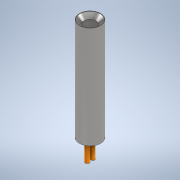
# Autodesk Inventor part: Heater630W
Saved by Autodesk Inventor 2020 (Build 240168000, 168)
## iProperties
Created: 2020-06-17
Part Number: Heater630W
Material: Steel, Alloy
Document SubType Name: Modeling
Designer: Juan
Density: 7.73 g/cm^3
Appearance: Semi-Polished
Author: Juan
Autodesk Inventor part; units mm, degrees
ref_plane "YZ Plane" through (0, 0, 0) normal (1, 0, 0) x (0, 1, 0)
ref_plane "XZ Plane" through (0, 0, 0) normal (0, 1, 0) x (-1, 0, 0)
ref_plane "XY Plane" through (0, 0, 0) normal (0, 0, 1) x (1, 0, 0)
sketch "Sketch1" plane through (0, 0, 0) normal (0, 1, 0) x (-1, 0, 0)
  circle A0 centre (0, 0) radius 7.9375
  dimension "d0" = 15.875
  constraints: 1 centre point, 1 coincident
  measures "d0" diameter of A0
extrude "Extrusion1" add sketch "Sketch1" along normal blind 76.2
sketch "Sketch2" plane through (0, 76.2, 0) normal (0, 1, 0) x (1, 0, 0)
  circle A0 centre (0, 0) radius 4.5
  dimension "d3" = 9
  constraints: 1 centre point, 1 coincident
  measures "d3" diameter of A0
extrude "Extrusion2" cut sketch "Sketch2" against normal blind 3
chamfer "Chamfer1" distance 3 angle 45 1 edges at (-4.5, 76.2, 0)
sketch "Sketch3" plane through (0, 0, 0) normal (0, -1, 0) x (1, 0, 0)
  circle A0 centre (0, 2) radius 1.5
  circle A1 centre (0, -2) radius 1.5
  point P0 (0, 0)
  dimension "d9" = 3
  dimension "d10" = 3
  dimension "d11" = 2
  dimension "d12" = 2
  constraints: 2 centre point, 2 vertical alignment
  measures "d9" diameter of A0
  measures "d10" diameter of A1
  measures "d11" distance of point (0, 0) A0.centre
  measures "d12" distance of point (0, 0) A1.centre
extrude "Extrusion3" add sketch "Sketch3" along normal blind 15
body "Solid1"
